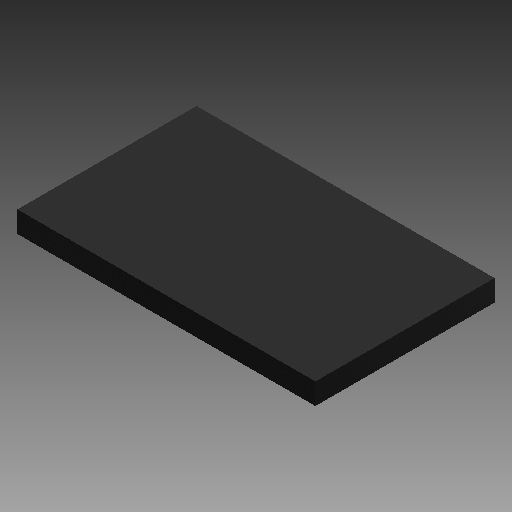
# Autodesk Inventor part: MONITOR
Saved by Autodesk Inventor 2017 SP1 (Build 210196100, 196)
## iProperties
Created: 2016-04-02
Part Number: MONITOR
Material: ABS Plastic
Document SubType Name: Modeling
Designer: hwasserb
Density: 1.06 g/cm^3
Appearance: Fine Textured - Black
Author: hwasserb
Autodesk Inventor part; units mm, degrees
ref_plane "YZ Plane" through (0, 0, 0) normal (1, 0, 0) x (0, 1, 0)
ref_plane "XZ Plane" through (0, 0, 0) normal (0, 1, 0) x (-1, 0, 0)
ref_plane "XY Plane" through (0, 0, 0) normal (0, 0, 1) x (1, 0, 0)
sketch "Sketch1" plane through (0, 0, 0) normal (0, 1, 0) x (-1, 0, 0)
  line L0 (0, 0) -> (533.4, 0)
  line L1 (533.4, 0) -> (533.4, -320.675)
  line L2 (533.4, -320.675) -> (0, -320.675)
  line L3 (0, -320.675) -> (0, 0)
  dimension "d0" = 533.4
  dimension "d1" = 320.675
  constraints: 8 end point, 2 parallel, 1 horizontal, 1 perpendicular
  measures "d0" distance of L0.start L0.end
  measures "d1" distance of L2.end L0.start
extrude "Extrusion1" add sketch "Sketch1" along normal blind 38.1
sketch "Sketch2" plane through (0, 0, 0) normal (0, -1, 0) x (1, 0, 0)
  line L0 (-533.4, 0) -> (-316.7, -98.425) construction
  line L1 (-216.7, -98.425) -> (0, 0) construction
  line L2 (0, 0) -> (-533.4, 0) projected
  point P0 (-316.7, -198.425)
  point P1 (-216.7, -198.425)
  dimension "d4" = 100
  dimension "d5" = 100
  dimension "d13" = 98.425
  constraints: 4 end point, 2 horizontal alignment, 2 vertical alignment, 1 equal length
  measures "d4" distance of L1.start L0.end
  measures "d5" distance of point (-216.7, -198.425) L1.start
  measures "d13" distance from line of L2 L1.start
hole "Hole1" at (-316.7, 0, -98.425) at (-216.7, 0, -98.425) at (-316.7, 0, -198.425) at (-216.7, 0, -198.425) direction (0, 1, 0) diameter 7 depth 12.7
body "Solid1"
